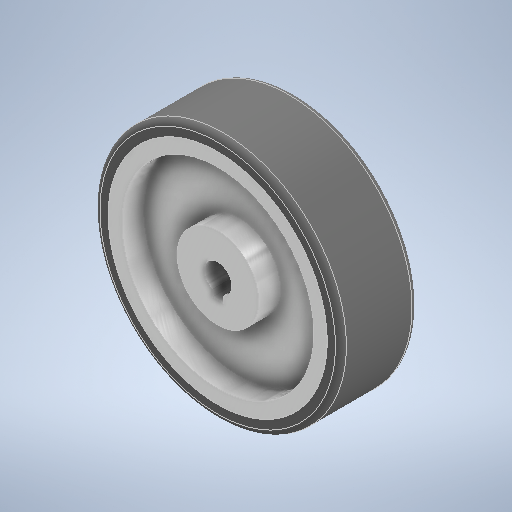
# Autodesk Inventor part: Part4
Saved by Autodesk Inventor 2025 (Build 290162000, 162)
## iProperties
Created: 2026-06-07
Part Number: Part4
Material: Generic
Document SubType Name: Modeling
Designer: user
Density: 1 g/cm^3
Appearance: Gray
Author: user
Autodesk Inventor part; units mm, degrees
ref_plane "YZ Plane" through (0, 0, 0) normal (1, 0, 0) x (0, 1, 0)
ref_plane "XZ Plane" through (0, 0, 0) normal (0, 1, 0) x (-1, 0, 0)
sketch "Sketch1" plane through (0, 0, 0) normal (0, 0, 1) x (1, 0, 0)
  circle A0 centre (0, 0) radius 40
  dimension "d0" = 80
  constraints: 1 centre point, 1 coincident
  measures "d0" diameter of A0
extrude "Extrusion1" add sketch "Sketch1" along normal blind 28
sketch "Sketch2" plane through (0, 0, 28) normal (0, 0, 1) x (1, 0, 0)
  circle A0 centre (0, 0) radius 35
  circle A1 centre (0, 0) radius 15
  dimension "d3" = 70
  dimension "d4" = 30
  constraints: 2 centre point, 2 coincident
  measures "d3" diameter of A0
  measures "d4" diameter of A1
extrude "Extrusion2" cut sketch "Sketch2" against normal blind 8
ref_plane "Work Plane1" through (0, 0, 14) normal (0, 0, 1) x (1, 0, 0)
mirror "Mirror1" about plane through (0, 0, 14) normal (0, 0, 1) of "Extrusion2"
sketch "Sketch3" plane through (0, 0, 0) normal (0, 0, -1) x (-1, 0, 0)
  circle A0 centre (0, 0) radius 5
  line L0 (0, -5) -> (0, -7)
  line L1 (0, -7) -> (-2, -7)
  line L2 (-2, -7) -> (-2, 0)
  line L3 (-2, 0) -> (2, 0)
  line L4 (2, 0) -> (2, -7)
  line L5 (2, -7) -> (0, -7)
  point P0 (2, -4.5826)
  point P1 (-2, -4.5826)
  dimension "d7" = 10
  dimension "d8" = 2
  dimension "d9" = 2
  dimension "d10" = 4
  constraints: 12 end point, 4 perpendicular, 1 coincident, 1 collinear, 1 point on line, 1 vertical, 3 other
  measures "d8" distance of L0.start L0.end
  measures "d9" distance of L0.end L1.end
  measures "d10" distance of L2.end L3.end
extrude "Extrusion3" cut sketch "Sketch3" against normal blind 30
sketch "Sketch4" plane through (0, 0, 0) normal (1, 0, 0) x (0, 1, 0)
  line L0 (40, 28) -> (-40, 28) projected
  line L1 (-40, 28) -> (-45, 28)
  line L2 (-45, 28) -> (-45, 0)
  line L3 (-45, 0) -> (-40, 0)
  line L4 (-40, 0) -> (-40, 28)
  line L5 (0, 28) -> (0, 0)
  line L6 (-4.5826, 0) -> (-4.5826, 28) projected
  dimension "d13" = 5
  constraints: 10 end point, 3 perpendicular, 1 horizontal, 1 midpoint, 1 parallel
  measures "d13" distance of L0.end L1.end
revolve "Revolution1" add sketch "Sketch4" angle 360 about axis through (0, 0, 28) along (0, 0, -1) separate body
fillet "Fillet1" radius 2 2 edges at (0, 45, 28) (0, 45, 0)
body "Solid1"
body "Solid2"
